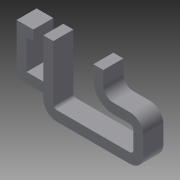
# Autodesk Inventor part: grapa
Saved by Autodesk Inventor 2015 (Build 190159000, 159)
## iProperties
Created: 2015-06-30
Part Number: grapa
Material: Genérico
Document SubType Name: Modeling
Designer: Roberto
Density: 1 g/cm^3
Appearance: Valor por defecto
Author: Roberto
Autodesk Inventor part; units mm, degrees
ref_plane "YZ Plane" through (0, 0, 0) normal (1, 0, 0) x (0, 1, 0)
ref_plane "XZ Plane" through (0, 0, 0) normal (0, 1, 0) x (-1, 0, 0)
ref_plane "XY Plane" through (0, 0, 0) normal (0, 0, 1) x (1, 0, 0)
sketch "Boceto1" plane through (0, 0, 0) normal (0, 1, 0) x (-1, 0, 0)
  line L0 (-63.5298, 15.6581) -> (-63.5298, 12.9581) projected
  line L1 (-51.5298, 15.6581) -> (-51.5298, 12.9581) projected
  line L2 (-52.0298, 12.4581) -> (-63.0298, 12.4581) projected
  line L3 (-51.5298, 17.1581) -> (-51.5298, 71.7081) projected
  line L4 (-57.5298, 69.7081) -> (-57.5298, 19.1581) projected
  line L5 (-63.0298, 16.1581) -> (-52.0298, 16.1581) projected
  arc A0 (-60.5298, 16.1581) -> (-57.5298, 19.1581) centre (-60.5298, 19.1581) ccw projected
  arc A1 (-63.0298, 16.1581) -> (-63.5298, 15.6581) centre (-63.0298, 15.6581) ccw projected
  arc A2 (-63.5298, 12.9581) -> (-63.0298, 12.4581) centre (-63.0298, 12.9581) ccw projected
  arc A3 (-52.0298, 12.4581) -> (-51.5298, 12.9581) centre (-52.0298, 12.9581) ccw projected
  line L6 (-51.5298, 15.6581) -> (-51.5298, 17.1581) projected
  line L7 (-60.5298, 17.6581) -> (-63.0298, 17.6581)
  arc A4 (-63.0298, 17.6581) -> (-65.0298, 15.6581) centre (-63.0298, 15.6581) ccw
  line L8 (-65.0298, 15.6581) -> (-65.0298, 12.9581)
  arc A5 (-65.0298, 12.9581) -> (-63.0298, 10.9581) centre (-63.0298, 12.9581) ccw
  line L9 (-63.0298, 10.9581) -> (-52.0298, 10.9581)
  arc A6 (-52.0298, 10.9581) -> (-50.0298, 12.9581) centre (-52.0298, 12.9581) ccw
  line L10 (-50.0298, 12.9581) -> (-50.0298, 15.6581)
  line L11 (-50.0298, 15.6581) -> (-50.0298, 17.1581)
  line L12 (-50.0298, 12.9581) -> (-50.0298, 21.1581)
  line L13 (-59.0298, 21.1581) -> (-59.0298, 19.1581)
  arc A7 (-60.5298, 17.6581) -> (-59.0298, 19.1581) centre (-60.5298, 19.1581) ccw
  line L14 (-59.0298, 21.1581) -> (-57.5298, 21.1581)
  line L15 (-50.0298, 21.1581) -> (-51.5298, 21.1581)
  line L16 (-51.5298, 21.1581) -> (-51.5298, 12.9581)
  line L17 (-52.0298, 12.4581) -> (-63.0298, 12.4581)
  line L18 (-63.5298, 12.9581) -> (-63.5298, 15.6581)
  line L19 (-63.0298, 16.1581) -> (-60.5298, 16.1581)
  line L20 (-57.5298, 21.1581) -> (-57.5298, 19.1581)
  line L21 (-57.5298, 21.1581) -> (-57.5298, 19.1581)
  arc A8 (-60.5298, 16.1581) -> (-57.5298, 19.1581) centre (-60.5298, 19.1581) ccw
  arc A9 (-63.0298, 16.1581) -> (-63.5298, 15.6581) centre (-63.0298, 15.6581) ccw
  arc A10 (-63.5298, 12.9581) -> (-63.0298, 12.4581) centre (-63.0298, 12.9581) ccw
  arc A11 (-52.0298, 12.4581) -> (-51.5298, 12.9581) centre (-52.0298, 12.9581) ccw
  line L22 (-50.0298, 13.6581) -> (-46.0298, 13.6581)
  line L23 (-46.0298, 13.6581) -> (-46.0298, 21.1581)
  line L24 (-47.5298, 15.1581) -> (-50.0298, 15.1581)
  line L25 (-46.0298, 21.1581) -> (-48.5298, 21.1581)
  line L26 (-48.5298, 21.1581) -> (-48.5298, 19.6581)
  line L27 (-47.5298, 15.1581) -> (-47.5298, 19.6581)
  line L28 (-47.5298, 19.6581) -> (-48.5298, 19.6581)
  point P0 (0, 0)
  dimension "d0" = 1.5
  dimension "d1" = 1.5
  dimension "d2" = 5
  dimension "d3" = 1.5
  dimension "d4" = 1.5
  dimension "d5" = 1.5
  dimension "d8" = 1.5
  dimension "d9" = 1.5
  dimension "d10" = 2.5
  dimension "d11" = 4
  dimension "d12" = 7.5
  constraints: 44 end point, 18 point on circle, 8 centre point, 8 point on line, 7 perpendicular, 4 collinear, 4 tangent, 1 concentric, 1 horizontal, 1 vertical, 6 other
  measures "d0" distance between parallel lines of L1 L10
  measures "d1" distance between parallel lines of L4 L13
  measures "d2" distance between parallel lines of L15 L5
  measures "d3" radius of A7
  measures "d4" distance between parallel lines of L5 L7
  measures "d5" distance between parallel lines of L22 L24
  measures "d8" distance between parallel lines of L23 L27
  measures "d9" distance of L25.end L26.end
  measures "d10" distance of L23.end L25.end
  measures "d11" distance of L22.start L22.end
  measures "d12" distance of L22.end L23.end
extrude "Extrusión1" add sketch "Boceto1" along normal blind 3
equation "\"d5\" = d0"
equation "\"d8\" = d0"
equation "\"d9\" = d0"
